ketchup (Autodesk Fusion 360 design; units mm, degrees)
Autodesk Fusion 360 part; units mm, degrees
sketch "Sketch1" plane through (0, 0, 0) normal (0, 0, 1) x (1, 0, 0)
  line L0 (0, 0) -> (-49, 0)
  line L1 (-49, 0) -> (-49, 88)
  line L2 (-49, 88) -> (0, 88)
  line L3 (0, 88) -> (0, 0)
  line L4 (-4, 4) -> (-45, 4)
  line L5 (-45, 4) -> (-45, 84)
  line L6 (-45, 84) -> (-4, 84)
  line L7 (-4, 84) -> (-4, 4)
  dimension "d1" = 49
  dimension "d2" = 88
  dimension "d3" = 4
  constraint horizontal L0
  constraint vertical L1
  constraint horizontal L2
  constraint vertical L3
  constraint coincident L0.start L3.end
  measures "d1" distance of L1.end L2.end
  measures "d2" distance of L0.start L2.end
extrude "Extrude1" add sketch "Sketch1" along normal blind 4 contours L0 L1 L2 L3 | L4 L5 L6 L7 makes body 1
extrude "Extrude2" add sketch "Sketch1" along normal blind 70 bodies 1
sketch "Sketch3" plane through (0, 0, 0) normal (0, -1, 0) x (1, 0, 0)
  line L0 (-49, 0) -> (0, 0)
  line L1 (0, 0) -> (0, 70)
  line L2 (0, 70) -> (-49, 70)
  line L3 (-49, 70) -> (-49, 0)
  line L4 (-43.8953, 12.2336) -> (-43.9282, 20.2336)
  line L5 (-43.9282, 20.2336) -> (-42.8695, 20.2379)
  line L6 (-42.8695, 20.2379) -> (-42.8532, 16.2707)
  line L7 (-42.8532, 16.2707) -> (-38.8968, 20.2542)
  line L8 (-38.8968, 20.2542) -> (-37.4617, 20.2601)
  line L9 (-37.4617, 20.2601) -> (-40.8044, 17.0049)
  line L10 (-40.8044, 17.0049) -> (-37.2815, 12.2608)
  line L11 (-37.2815, 12.2608) -> (-38.6784, 12.2551)
  line L12 (-38.6784, 12.2551) -> (-41.5436, 16.2924)
  line L13 (-41.5436, 16.2924) -> (-42.848, 15.0101)
  line L14 (-42.848, 15.0101) -> (-42.8367, 12.238)
  line L15 (-42.8367, 12.238) -> (-43.8953, 12.2336)
  line L16 (-32.5634, 14.1465) -> (-31.5479, 14.0252)
  spline S0 degree 2 poles (-31.5479, 14.0252) (-31.7843, 13.1347) (-32.4317, 12.6409) knots 0 0 0 1 1 1
  spline S1 degree 2 poles (-32.4317, 12.6409) (-33.079, 12.1471) (-34.0886, 12.143) knots 0 0 0 1 1 1
  spline S2 degree 2 poles (-34.0886, 12.143) (-35.3601, 12.1377) (-36.1082, 12.9178) knots 0 0 0 1 1 1
  spline S3 degree 2 poles (-36.1082, 12.9178) (-36.8562, 13.6978) (-36.8621, 15.1111) knots 0 0 0 1 1 1
  spline S4 degree 2 poles (-36.8621, 15.1111) (-36.8681, 16.5736) (-36.1183, 17.3843) knots 0 0 0 1 1 1
  spline S5 degree 2 poles (-36.1183, 17.3843) (-35.3686, 18.195) (-34.168, 18.2) knots 0 0 0 1 1 1
  spline S6 degree 2 poles (-34.168, 18.2) (-33.0057, 18.2048) (-32.2658, 17.4165) knots 0 0 0 1 1 1
  spline S7 degree 2 poles (-32.2658, 17.4165) (-31.5258, 16.6283) (-31.5199, 15.1931) knots 0 0 0 1 1 1
  spline S8 degree 2 poles (-31.5199, 15.1931) (-31.5196, 15.1058) (-31.5243, 14.9311) knots 0 0 0 1 1 1
  line L17 (-31.5243, 14.9311) -> (-35.8462, 14.9134)
  spline S9 degree 2 poles (-35.8462, 14.9134) (-35.7877, 13.9586) (-35.3, 13.4531) knots 0 0 0 1 1 1
  spline S10 degree 2 poles (-35.3, 13.4531) (-34.8122, 12.9476) (-34.0864, 12.9506) knots 0 0 0 1 1 1
  spline S11 degree 2 poles (-34.0864, 12.9506) (-33.5462, 12.9528) (-33.1654, 13.2382) knots 0 0 0 1 1 1
  spline S12 degree 2 poles (-33.1654, 13.2382) (-32.7846, 13.5235) (-32.5634, 14.1465) knots 0 0 0 1 1 1
  line L18 (-35.795, 15.7212) -> (-32.559, 15.7345)
  spline S13 degree 2 poles (-32.559, 15.7345) (-32.6275, 16.4655) (-32.9346, 16.8299) knots 0 0 0 1 1 1
  spline S14 degree 2 poles (-32.9346, 16.8299) (-33.4062, 17.3955) (-34.1538, 17.3924) knots 0 0 0 1 1 1
  spline S15 degree 2 poles (-34.1538, 17.3924) (-34.8305, 17.3896) (-35.2897, 16.9348) knots 0 0 0 1 1 1
  spline S16 degree 2 poles (-35.2897, 16.9348) (-35.749, 16.48) (-35.795, 15.7212) knots 0 0 0 1 1 1
  line L19 (-28.1664, 13.1768) -> (-28.021, 12.3098)
  spline S17 degree 2 poles (-28.021, 12.3098) (-28.4354, 12.2208) (-28.7628, 12.2194) knots 0 0 0 1 1 1
  spline S18 degree 2 poles (-28.7628, 12.2194) (-29.2976, 12.2172) (-29.5929, 12.3852) knots 0 0 0 1 1 1
  spline S19 degree 2 poles (-29.5929, 12.3852) (-29.8883, 12.5531) (-30.0095, 12.8282) knots 0 0 0 1 1 1
  spline S20 degree 2 poles (-30.0095, 12.8282) (-30.1307, 13.1033) (-30.1343, 13.9873) knots 0 0 0 1 1 1
  line L20 (-30.1343, 13.9873) -> (-30.148, 17.3215)
  line L21 (-30.148, 17.3215) -> (-30.8683, 17.3186)
  line L22 (-30.8683, 17.3186) -> (-30.8715, 18.0826)
  line L23 (-30.8715, 18.0826) -> (-30.1512, 18.0855)
  line L24 (-30.1512, 18.0855) -> (-30.1571, 19.5207)
  line L25 (-30.1571, 19.5207) -> (-29.1827, 20.1141)
  line L26 (-29.1827, 20.1141) -> (-29.1744, 18.0895)
  line L27 (-29.1744, 18.0895) -> (-28.1866, 18.0936)
  line L28 (-28.1866, 18.0936) -> (-28.1835, 17.3296)
  line L29 (-28.1835, 17.3296) -> (-29.1712, 17.3256)
  line L30 (-29.1712, 17.3256) -> (-29.1573, 13.9368)
  spline S21 degree 2 poles (-29.1573, 13.9368) (-29.1556, 13.5166) (-29.1032, 13.3967) knots 0 0 0 1 1 1
  spline S22 degree 2 poles (-29.1032, 13.3967) (-29.0509, 13.2769) (-28.9333, 13.2064) knots 0 0 0 1 1 1
  spline S23 degree 2 poles (-28.9333, 13.2064) (-28.8157, 13.136) (-28.5974, 13.1369) knots 0 0 0 1 1 1
  spline S24 degree 2 poles (-28.5974, 13.1369) (-28.4337, 13.1375) (-28.1664, 13.1768) knots 0 0 0 1 1 1
  line L31 (-23.4294, 14.4405) -> (-22.463, 14.319)
  spline S25 degree 2 poles (-22.463, 14.319) (-22.6172, 13.3197) (-23.267, 12.7522) knots 0 0 0 1 1 1
  spline S26 degree 2 poles (-23.267, 12.7522) (-23.9168, 12.1847) (-24.8663, 12.1808) knots 0 0 0 1 1 1
  spline S27 degree 2 poles (-24.8663, 12.1808) (-26.0559, 12.176) (-26.7821, 12.9506) knots 0 0 0 1 1 1
  spline S28 degree 2 poles (-26.7821, 12.9506) (-27.5084, 13.7253) (-27.5144, 15.1768) knots 0 0 0 1 1 1
  spline S29 degree 2 poles (-27.5144, 15.1768) (-27.5182, 16.1154) (-27.2101, 16.8206) knots 0 0 0 1 1 1
  spline S30 degree 2 poles (-27.2101, 16.8206) (-26.9019, 17.5259) (-26.2676, 17.8805) knots 0 0 0 1 1 1
  spline S31 degree 2 poles (-26.2676, 17.8805) (-25.6333, 18.235) (-24.8857, 18.2381) knots 0 0 0 1 1 1
  spline S32 degree 2 poles (-24.8857, 18.2381) (-23.9417, 18.242) (-23.3394, 17.767) knots 0 0 0 1 1 1
  spline S33 degree 2 poles (-23.3394, 17.767) (-22.7372, 17.292) (-22.5644, 16.4141) knots 0 0 0 1 1 1
  line L32 (-22.5644, 16.4141) -> (-23.5188, 16.2628)
  spline S34 degree 2 poles (-23.5188, 16.2628) (-23.6576, 16.8462) (-24.0053, 17.1394) knots 0 0 0 1 1 1
  spline S35 degree 2 poles (-24.0053, 17.1394) (-24.3531, 17.4327) (-24.8442, 17.4306) knots 0 0 0 1 1 1
  spline S36 degree 2 poles (-24.8442, 17.4306) (-25.5863, 17.4276) (-26.048, 16.8936) knots 0 0 0 1 1 1
  spline S37 degree 2 poles (-26.048, 16.8936) (-26.5097, 16.3597) (-26.5049, 15.2082) knots 0 0 0 1 1 1
  spline S38 degree 2 poles (-26.5049, 15.2082) (-26.5001, 14.0405) (-26.0505, 13.513) knots 0 0 0 1 1 1
  spline S39 degree 2 poles (-26.0505, 13.513) (-25.6008, 12.9855) (-24.8805, 12.9884) knots 0 0 0 1 1 1
  spline S40 degree 2 poles (-24.8805, 12.9884) (-24.3021, 12.9908) (-23.9161, 13.3471) knots 0 0 0 1 1 1
  spline S41 degree 2 poles (-23.9161, 13.3471) (-23.5301, 13.7034) (-23.4294, 14.4405) knots 0 0 0 1 1 1
  line L33 (-21.6145, 12.3252) -> (-21.6473, 20.3251)
  line L34 (-21.6473, 20.3251) -> (-20.6651, 20.3291)
  line L35 (-20.6651, 20.3291) -> (-20.6533, 17.4588)
  spline S42 degree 2 poles (-20.6533, 17.4588) (-19.969, 18.2583) (-18.9212, 18.2626) knots 0 0 0 1 1 1
  spline S43 degree 2 poles (-18.9212, 18.2626) (-18.2773, 18.2653) (-17.8015, 18.0135) knots 0 0 0 1 1 1
  spline S44 degree 2 poles (-17.8015, 18.0135) (-17.3257, 17.7617) (-17.1192, 17.315) knots 0 0 0 1 1 1
  spline S45 degree 2 poles (-17.1192, 17.315) (-16.9128, 16.8684) (-16.9093, 16.0171) knots 0 0 0 1 1 1
  line L36 (-16.9093, 16.0171) -> (-16.8942, 12.3446)
  line L37 (-16.8942, 12.3446) -> (-17.8764, 12.3405)
  line L38 (-17.8764, 12.3405) -> (-17.8915, 16.0131)
  spline S46 degree 2 poles (-17.8915, 16.0131) (-17.8945, 16.7498) (-18.2152, 17.0841) knots 0 0 0 1 1 1
  spline S47 degree 2 poles (-18.2152, 17.0841) (-18.5358, 17.4184) (-19.1197, 17.416) knots 0 0 0 1 1 1
  spline S48 degree 2 poles (-19.1197, 17.416) (-19.5562, 17.4142) (-19.94, 17.1861) knots 0 0 0 1 1 1
  spline S49 degree 2 poles (-19.94, 17.1861) (-20.3238, 16.9581) (-20.4859, 16.57) knots 0 0 0 1 1 1
  spline S50 degree 2 poles (-20.4859, 16.57) (-20.648, 16.1818) (-20.6452, 15.4997) knots 0 0 0 1 1 1
  line L39 (-20.6452, 15.4997) -> (-20.6322, 12.3292)
  line L40 (-20.6322, 12.3292) -> (-21.6145, 12.3252)
  line L41 (-11.6009, 12.3663) -> (-11.6044, 13.2176)
  spline S51 degree 2 poles (-11.6044, 13.2176) (-12.277, 12.2326) (-13.4394, 12.2278) knots 0 0 0 1 1 1
  spline S52 degree 2 poles (-13.4394, 12.2278) (-13.9523, 12.2257) (-14.3979, 12.4203) knots 0 0 0 1 1 1
  spline S53 degree 2 poles (-14.3979, 12.4203) (-14.8434, 12.6149) (-15.0602, 12.9115) knots 0 0 0 1 1 1
  spline S54 degree 2 poles (-15.0602, 12.9115) (-15.277, 13.208) (-15.3661, 13.6387) knots 0 0 0 1 1 1
  spline S55 degree 2 poles (-15.3661, 13.6387) (-15.4273, 13.9277) (-15.4298, 14.5552) knots 0 0 0 1 1 1
  line L42 (-15.4298, 14.5552) -> (-15.4446, 18.1459)
  line L43 (-15.4446, 18.1459) -> (-14.4623, 18.15)
  line L44 (-14.4623, 18.15) -> (-14.4491, 14.9358)
  spline S56 degree 2 poles (-14.4491, 14.9358) (-14.446, 14.1664) (-14.3849, 13.8992) knots 0 0 0 1 1 1
  spline S57 degree 2 poles (-14.3849, 13.8992) (-14.2905, 13.5122) (-13.9894, 13.2924) knots 0 0 0 1 1 1
  spline S58 degree 2 poles (-13.9894, 13.2924) (-13.6884, 13.0726) (-13.2464, 13.0744) knots 0 0 0 1 1 1
  spline S59 degree 2 poles (-13.2464, 13.0744) (-12.8044, 13.0762) (-12.4179, 13.3043) knots 0 0 0 1 1 1
  spline S60 degree 2 poles (-12.4179, 13.3043) (-12.0313, 13.5324) (-11.872, 13.9232) knots 0 0 0 1 1 1
  spline S61 degree 2 poles (-11.872, 13.9232) (-11.7126, 14.314) (-11.7156, 15.0562) knots 0 0 0 1 1 1
  line L45 (-11.7156, 15.0562) -> (-11.7284, 18.1612)
  line L46 (-11.7284, 18.1612) -> (-10.7461, 18.1652)
  line L47 (-10.7461, 18.1652) -> (-10.7223, 12.3699)
  line L48 (-10.7223, 12.3699) -> (-11.6009, 12.3663)
  line L49 (-9.1743, 10.1553) -> (-9.2073, 18.1716)
  line L50 (-9.2073, 18.1716) -> (-8.3123, 18.1752)
  line L51 (-8.3123, 18.1752) -> (-8.3092, 17.4222)
  spline S62 degree 2 poles (-8.3092, 17.4222) (-7.9945, 17.8655) (-7.5971, 18.0881) knots 0 0 0 1 1 1
  spline S63 degree 2 poles (-7.5971, 18.0881) (-7.1996, 18.3108) (-6.6321, 18.3131) knots 0 0 0 1 1 1
  spline S64 degree 2 poles (-6.6321, 18.3131) (-5.89, 18.3162) (-5.3209, 17.9365) knots 0 0 0 1 1 1
  spline S65 degree 2 poles (-5.3209, 17.9365) (-4.7518, 17.5568) (-4.4597, 16.8623) knots 0 0 0 1 1 1
  spline S66 degree 2 poles (-4.4597, 16.8623) (-4.1676, 16.1677) (-4.1642, 15.3382) knots 0 0 0 1 1 1
  spline S67 degree 2 poles (-4.1642, 15.3382) (-4.1606, 14.4487) (-4.4769, 13.7353) knots 0 0 0 1 1 1
  spline S68 degree 2 poles (-4.4769, 13.7353) (-4.7932, 13.0218) (-5.4001, 12.6401) knots 0 0 0 1 1 1
  spline S69 degree 2 poles (-5.4001, 12.6401) (-6.007, 12.2583) (-6.6782, 12.2556) knots 0 0 0 1 1 1
  spline S70 degree 2 poles (-6.6782, 12.2556) (-7.1693, 12.2536) (-7.5603, 12.4593) knots 0 0 0 1 1 1
  spline S71 degree 2 poles (-7.5603, 12.4593) (-7.9514, 12.6651) (-8.2037, 12.9806) knots 0 0 0 1 1 1
  line L52 (-8.2037, 12.9806) -> (-8.1921, 10.1593)
  line L53 (-8.1921, 10.1593) -> (-9.1743, 10.1553)
  spline S72 degree 2 poles (-8.3057, 15.2448) (-8.3011, 14.1261) (-7.846, 13.5932) knots 0 0 0 1 1 1
  spline S73 degree 2 poles (-7.846, 13.5932) (-7.3909, 13.0603) (-6.747, 13.0629) knots 0 0 0 1 1 1
  spline S74 degree 2 poles (-6.747, 13.0629) (-6.0921, 13.0656) (-5.6278, 13.6214) knots 0 0 0 1 1 1
  spline S75 degree 2 poles (-5.6278, 13.6214) (-5.1635, 14.1772) (-5.1683, 15.3396) knots 0 0 0 1 1 1
  spline S76 degree 2 poles (-5.1683, 15.3396) (-5.1729, 16.4473) (-5.6308, 16.9966) knots 0 0 0 1 1 1
  spline S77 degree 2 poles (-5.6308, 16.9966) (-6.0887, 17.5459) (-6.7217, 17.5433) knots 0 0 0 1 1 1
  spline S78 degree 2 poles (-6.7217, 17.5433) (-7.3493, 17.5407) (-7.8298, 16.9521) knots 0 0 0 1 1 1
  spline S79 degree 2 poles (-7.8298, 16.9521) (-8.3103, 16.3635) (-8.3057, 15.2448) knots 0 0 0 1 1 1
extrude "Extrude3" cut sketch "Sketch3" against normal blind 1 contours L4 L5 L6 L7 L8 L9 L10 L11 L12 L13 L14 L15 | L16 S0 S1 S2 S3 S4 S5 S6 S7 S8 L17 S9 S10 S11 S12 | L19 S17 S18 S19 S20 L20 L21 L22 L23 L24 L25 L26 L27 L28 L29 L30 S21 S22 S23 S24 | L31 S25 S26 S27 S28 S29 S30 S31 S32 S33 L32 S34 S35 S36 S37 S38 S39 S40 S41 | L33 L34 L35 S42 S43 S44 S45 L36 L37 L38 S46 S47 S48 S49 S50 L39 L40 | L41 S51 S52 S53 S54 S55 L42 L43 L44 S56 S57 S58 S59 S60 S61 L45 L46 L47 L48 | L49 L50 L51 S62 S63 S64 S65 S66 S67 S68 S69 S70 S71 L52 L53 bodies 1
sketch "Sketch5" plane through (0, 0, 70) normal (0, 0, 1) x (-1, 0, 0)
  line L0 (45, -84) -> (4, -84)
  line L1 (4, -84) -> (4, -4)
  line L2 (4, -4) -> (45, -4)
  line L3 (45, -4) -> (45, -84)
  line L4 (0, -88) -> (49, -88)
  line L5 (49, -88) -> (49, 0)
  line L6 (49, 0) -> (0, 0)
  line L7 (0, 0) -> (0, -88)
  line L8 (4, -4) -> (4, 0)
  line L9 (45, -4) -> (45, 0)
  constraint coincident L1.end L2.start
  constraint coincident L6 L8.end
  constraint perpendicular L6 L8
  constraint coincident L2.end L3.start
  constraint coincident L6 L9.end
  constraint perpendicular L6 L9
sketch "Sketch4" plane through (0, 0, 0) normal (0, -1, 0) x (1, 0, 0)
  line L0 (-49, 0) -> (0, 0)
  line L1 (0, 0) -> (0, 70)
  line L2 (0, 70) -> (-49, 70)
  line L3 (-49, 70) -> (-49, 0)
  spline S0 degree 2 poles (-45, 70) (-24.5, 0) (-4, 70) knots 0 0 0 8.378065 8.378065 8.378065 weights 1 1.091518 1
  line L4 (-24.5, 0) -> (-24.5, 70)
  spline S1 degree 2 poles (-20.4859, 16.57) (-20.648, 16.1818) (-20.6452, 15.4997) knots 0 0 0 1 1 1
  line L5 (-20.6452, 15.4997) -> (-20.6322, 12.3292)
  line L6 (-20.6322, 12.3292) -> (-21.6145, 12.3252)
  line L7 (-21.6145, 12.3252) -> (-21.6473, 20.3251)
  line L8 (-21.6473, 20.3251) -> (-20.6651, 20.3291)
  line L9 (-20.6651, 20.3291) -> (-20.6533, 17.4588)
  spline S2 degree 2 poles (-20.6533, 17.4588) (-19.969, 18.2583) (-18.9212, 18.2626) knots 0 0 0 1 1 1
  spline S3 degree 2 poles (-18.9212, 18.2626) (-18.2773, 18.2653) (-17.8015, 18.0135) knots 0 0 0 1 1 1
  spline S4 degree 2 poles (-17.8015, 18.0135) (-17.3257, 17.7617) (-17.1192, 17.315) knots 0 0 0 1 1 1
  spline S5 degree 2 poles (-17.1192, 17.315) (-16.9128, 16.8684) (-16.9093, 16.0171) knots 0 0 0 1 1 1
  line L10 (-16.9093, 16.0171) -> (-16.8942, 12.3446)
  line L11 (-16.8942, 12.3446) -> (-17.8764, 12.3405)
  line L12 (-17.8764, 12.3405) -> (-17.8915, 16.0131)
  spline S6 degree 2 poles (-17.8915, 16.0131) (-17.8945, 16.7498) (-18.2152, 17.0841) knots 0 0 0 1 1 1
  spline S7 degree 2 poles (-18.2152, 17.0841) (-18.5358, 17.4184) (-19.1197, 17.416) knots 0 0 0 1 1 1
  spline S8 degree 2 poles (-19.1197, 17.416) (-19.5562, 17.4142) (-19.94, 17.1861) knots 0 0 0 1 1 1
  spline S9 degree 2 poles (-19.94, 17.1861) (-20.3238, 16.9581) (-20.4859, 16.57) knots 0 0 0 1 1 1
  line L13 (-41.5436, 16.2924) -> (-42.848, 15.0101)
  line L14 (-42.848, 15.0101) -> (-42.8367, 12.238)
  line L15 (-42.8367, 12.238) -> (-43.8953, 12.2336)
  line L16 (-43.8953, 12.2336) -> (-43.9282, 20.2336)
  line L17 (-43.9282, 20.2336) -> (-42.8695, 20.2379)
  line L18 (-42.8695, 20.2379) -> (-42.8532, 16.2707)
  line L19 (-42.8532, 16.2707) -> (-38.8968, 20.2542)
  line L20 (-38.8968, 20.2542) -> (-37.4617, 20.2601)
  line L21 (-37.4617, 20.2601) -> (-40.8044, 17.0049)
  line L22 (-40.8044, 17.0049) -> (-37.2815, 12.2608)
  line L23 (-37.2815, 12.2608) -> (-38.6784, 12.2551)
  line L24 (-38.6784, 12.2551) -> (-41.5436, 16.2924)
  spline S10 degree 2 poles (-26.0505, 13.513) (-25.6008, 12.9855) (-24.8805, 12.9884) knots 0 0 0 1 1 1
  spline S11 degree 2 poles (-24.8805, 12.9884) (-24.3021, 12.9908) (-23.9161, 13.3471) knots 0 0 0 1 1 1
  spline S12 degree 2 poles (-23.9161, 13.3471) (-23.5301, 13.7034) (-23.4294, 14.4405) knots 0 0 0 1 1 1
  line L25 (-23.4294, 14.4405) -> (-22.463, 14.319)
  spline S13 degree 2 poles (-22.463, 14.319) (-22.6172, 13.3197) (-23.267, 12.7522) knots 0 0 0 1 1 1
  spline S14 degree 2 poles (-23.267, 12.7522) (-23.9168, 12.1847) (-24.8663, 12.1808) knots 0 0 0 1 1 1
  spline S15 degree 2 poles (-24.8663, 12.1808) (-26.0559, 12.176) (-26.7821, 12.9506) knots 0 0 0 1 1 1
  spline S16 degree 2 poles (-26.7821, 12.9506) (-27.5084, 13.7253) (-27.5144, 15.1768) knots 0 0 0 1 1 1
  spline S17 degree 2 poles (-27.5144, 15.1768) (-27.5182, 16.1154) (-27.2101, 16.8206) knots 0 0 0 1 1 1
  spline S18 degree 2 poles (-27.2101, 16.8206) (-26.9019, 17.5259) (-26.2676, 17.8805) knots 0 0 0 1 1 1
  spline S19 degree 2 poles (-26.2676, 17.8805) (-25.6333, 18.235) (-24.8857, 18.2381) knots 0 0 0 1 1 1
  spline S20 degree 2 poles (-24.8857, 18.2381) (-23.9417, 18.242) (-23.3394, 17.767) knots 0 0 0 1 1 1
  spline S21 degree 2 poles (-23.3394, 17.767) (-22.7372, 17.292) (-22.5644, 16.4141) knots 0 0 0 1 1 1
  line L26 (-22.5644, 16.4141) -> (-23.5188, 16.2628)
  spline S22 degree 2 poles (-23.5188, 16.2628) (-23.6576, 16.8462) (-24.0053, 17.1394) knots 0 0 0 1 1 1
  spline S23 degree 2 poles (-24.0053, 17.1394) (-24.3531, 17.4327) (-24.8442, 17.4306) knots 0 0 0 1 1 1
  spline S24 degree 2 poles (-24.8442, 17.4306) (-25.5863, 17.4276) (-26.048, 16.8936) knots 0 0 0 1 1 1
  spline S25 degree 2 poles (-26.048, 16.8936) (-26.5097, 16.3597) (-26.5049, 15.2082) knots 0 0 0 1 1 1
  spline S26 degree 2 poles (-26.5049, 15.2082) (-26.5001, 14.0405) (-26.0505, 13.513) knots 0 0 0 1 1 1
  line L27 (-11.7284, 18.1612) -> (-10.7461, 18.1652)
  line L28 (-10.7461, 18.1652) -> (-10.7223, 12.3699)
  line L29 (-10.7223, 12.3699) -> (-11.6009, 12.3663)
  line L30 (-11.6009, 12.3663) -> (-11.6044, 13.2176)
  spline S27 degree 2 poles (-11.6044, 13.2176) (-12.277, 12.2326) (-13.4394, 12.2278) knots 0 0 0 1 1 1
  spline S28 degree 2 poles (-13.4394, 12.2278) (-13.9523, 12.2257) (-14.3979, 12.4203) knots 0 0 0 1 1 1
  spline S29 degree 2 poles (-14.3979, 12.4203) (-14.8434, 12.6149) (-15.0602, 12.9115) knots 0 0 0 1 1 1
  spline S30 degree 2 poles (-15.0602, 12.9115) (-15.277, 13.208) (-15.3661, 13.6387) knots 0 0 0 1 1 1
  spline S31 degree 2 poles (-15.3661, 13.6387) (-15.4273, 13.9277) (-15.4298, 14.5552) knots 0 0 0 1 1 1
  line L31 (-15.4298, 14.5552) -> (-15.4446, 18.1459)
  line L32 (-15.4446, 18.1459) -> (-14.4623, 18.15)
  line L33 (-14.4623, 18.15) -> (-14.4491, 14.9358)
  spline S32 degree 2 poles (-14.4491, 14.9358) (-14.446, 14.1664) (-14.3849, 13.8992) knots 0 0 0 1 1 1
  spline S33 degree 2 poles (-14.3849, 13.8992) (-14.2905, 13.5122) (-13.9894, 13.2924) knots 0 0 0 1 1 1
  spline S34 degree 2 poles (-13.9894, 13.2924) (-13.6884, 13.0726) (-13.2464, 13.0744) knots 0 0 0 1 1 1
  spline S35 degree 2 poles (-13.2464, 13.0744) (-12.8044, 13.0762) (-12.4179, 13.3043) knots 0 0 0 1 1 1
  spline S36 degree 2 poles (-12.4179, 13.3043) (-12.0313, 13.5324) (-11.872, 13.9232) knots 0 0 0 1 1 1
  spline S37 degree 2 poles (-11.872, 13.9232) (-11.7126, 14.314) (-11.7156, 15.0562) knots 0 0 0 1 1 1
  line L34 (-11.7156, 15.0562) -> (-11.7284, 18.1612)
  spline S38 degree 2 poles (-35.3, 13.4531) (-34.8122, 12.9476) (-34.0864, 12.9506) knots 0 0 0 1 1 1
  spline S39 degree 2 poles (-34.0864, 12.9506) (-33.5462, 12.9528) (-33.1654, 13.2382) knots 0 0 0 1 1 1
  spline S40 degree 2 poles (-33.1654, 13.2382) (-32.7846, 13.5235) (-32.5634, 14.1465) knots 0 0 0 1 1 1
  line L35 (-32.5634, 14.1465) -> (-31.5479, 14.0252)
  spline S41 degree 2 poles (-31.5479, 14.0252) (-31.7843, 13.1347) (-32.4317, 12.6409) knots 0 0 0 1 1 1
  spline S42 degree 2 poles (-32.4317, 12.6409) (-33.079, 12.1471) (-34.0886, 12.143) knots 0 0 0 1 1 1
  spline S43 degree 2 poles (-34.0886, 12.143) (-35.3601, 12.1377) (-36.1082, 12.9178) knots 0 0 0 1 1 1
  spline S44 degree 2 poles (-36.1082, 12.9178) (-36.8562, 13.6978) (-36.8621, 15.1111) knots 0 0 0 1 1 1
  spline S45 degree 2 poles (-36.8621, 15.1111) (-36.8681, 16.5736) (-36.1183, 17.3843) knots 0 0 0 1 1 1
  spline S46 degree 2 poles (-36.1183, 17.3843) (-35.3686, 18.195) (-34.168, 18.2) knots 0 0 0 1 1 1
  spline S47 degree 2 poles (-34.168, 18.2) (-33.0057, 18.2048) (-32.2658, 17.4165) knots 0 0 0 1 1 1
  spline S48 degree 2 poles (-32.2658, 17.4165) (-31.5258, 16.6283) (-31.5199, 15.1931) knots 0 0 0 1 1 1
  spline S49 degree 2 poles (-31.5199, 15.1931) (-31.5196, 15.1058) (-31.5243, 14.9311) knots 0 0 0 1 1 1
  line L36 (-31.5243, 14.9311) -> (-35.8462, 14.9134)
  spline S50 degree 2 poles (-35.8462, 14.9134) (-35.7877, 13.9586) (-35.3, 13.4531) knots 0 0 0 1 1 1
  spline S51 degree 2 poles (-29.1032, 13.3967) (-29.0509, 13.2769) (-28.9333, 13.2064) knots 0 0 0 1 1 1
  spline S52 degree 2 poles (-28.9333, 13.2064) (-28.8157, 13.136) (-28.5974, 13.1369) knots 0 0 0 1 1 1
  spline S53 degree 2 poles (-28.5974, 13.1369) (-28.4337, 13.1375) (-28.1664, 13.1768) knots 0 0 0 1 1 1
  line L37 (-28.1664, 13.1768) -> (-28.021, 12.3098)
  spline S54 degree 2 poles (-28.021, 12.3098) (-28.4354, 12.2208) (-28.7628, 12.2194) knots 0 0 0 1 1 1
  spline S55 degree 2 poles (-28.7628, 12.2194) (-29.2976, 12.2172) (-29.5929, 12.3852) knots 0 0 0 1 1 1
  spline S56 degree 2 poles (-29.5929, 12.3852) (-29.8883, 12.5531) (-30.0095, 12.8282) knots 0 0 0 1 1 1
  spline S57 degree 2 poles (-30.0095, 12.8282) (-30.1307, 13.1033) (-30.1343, 13.9873) knots 0 0 0 1 1 1
  line L38 (-30.1343, 13.9873) -> (-30.148, 17.3215)
  line L39 (-30.148, 17.3215) -> (-30.8683, 17.3186)
  line L40 (-30.8683, 17.3186) -> (-30.8715, 18.0826)
  line L41 (-30.8715, 18.0826) -> (-30.1512, 18.0855)
  line L42 (-30.1512, 18.0855) -> (-30.1571, 19.5207)
  line L43 (-30.1571, 19.5207) -> (-29.1827, 20.1141)
  line L44 (-29.1827, 20.1141) -> (-29.1744, 18.0895)
  line L45 (-29.1744, 18.0895) -> (-28.1866, 18.0936)
  line L46 (-28.1866, 18.0936) -> (-28.1835, 17.3296)
  line L47 (-28.1835, 17.3296) -> (-29.1712, 17.3256)
  line L48 (-29.1712, 17.3256) -> (-29.1573, 13.9368)
  spline S58 degree 2 poles (-29.1573, 13.9368) (-29.1556, 13.5166) (-29.1032, 13.3967) knots 0 0 0 1 1 1
  spline S59 degree 2 poles (-7.5603, 12.4593) (-7.9514, 12.6651) (-8.2037, 12.9806) knots 0 0 0 1 1 1
  line L49 (-8.2037, 12.9806) -> (-8.1921, 10.1593)
  line L50 (-8.1921, 10.1593) -> (-9.1743, 10.1553)
  line L51 (-9.1743, 10.1553) -> (-9.2073, 18.1716)
  line L52 (-9.2073, 18.1716) -> (-8.3123, 18.1752)
  line L53 (-8.3123, 18.1752) -> (-8.3092, 17.4222)
  spline S60 degree 2 poles (-8.3092, 17.4222) (-7.9945, 17.8655) (-7.5971, 18.0881) knots 0 0 0 1 1 1
  spline S61 degree 2 poles (-7.5971, 18.0881) (-7.1996, 18.3108) (-6.6321, 18.3131) knots 0 0 0 1 1 1
  spline S62 degree 2 poles (-6.6321, 18.3131) (-5.89, 18.3162) (-5.3209, 17.9365) knots 0 0 0 1 1 1
  spline S63 degree 2 poles (-5.3209, 17.9365) (-4.7518, 17.5568) (-4.4597, 16.8623) knots 0 0 0 1 1 1
  spline S64 degree 2 poles (-4.4597, 16.8623) (-4.1676, 16.1677) (-4.1642, 15.3382) knots 0 0 0 1 1 1
  spline S65 degree 2 poles (-4.1642, 15.3382) (-4.1606, 14.4487) (-4.4769, 13.7353) knots 0 0 0 1 1 1
  spline S66 degree 2 poles (-4.4769, 13.7353) (-4.7932, 13.0218) (-5.4001, 12.6401) knots 0 0 0 1 1 1
  spline S67 degree 2 poles (-5.4001, 12.6401) (-6.007, 12.2583) (-6.6782, 12.2556) knots 0 0 0 1 1 1
  spline S68 degree 2 poles (-6.6782, 12.2556) (-7.1693, 12.2536) (-7.5603, 12.4593) knots 0 0 0 1 1 1
  point P0 (-4, 70)
  point P1 (-45, 70)
  constraint coincident L2 P0
  constraint coincident L2 P1
  constraint coincident P0 S0.end
  constraint coincident P1 S0.start
  constraint midpoint L0 L4.start
  constraint midpoint L2 L4.end
extrude "Extrude4" cut sketch "Sketch4" against normal blind 66 contours L2 S0 L4 | L2 S0 L4 bodies 1
extrude "Extrude1'" add 7 faces at (-38.9214, 1, 13.8403) (-33.3098, 1, 15.193) (-29.4876, 1, 15.0832) (-26.8229, 1, 14.866) (-21.2999, 1, 16.1494) (-11.0614, 1, 15.1971) (-8.8813, 1, 14.3177) along direction (0, -1, 0) blind 1 separate body on bodies 1 makes body 2 at (-11.0614, 1, 15.1971) makes body 3 at (-26.8229, 1, 14.866) makes body 4 at (-33.3098, 1, 15.193) makes body 5 at (-38.9214, 1, 13.8403) makes body 6 at (-29.4876, 1, 15.0832) makes body 7 at (-21.2999, 1, 16.1494) makes body 8 at (-8.8813, 1, 14.3177) in component "Component"
component "Component" placed x (1, 0, 0) y (0, 1, 0) z (0, 0, 1) at (0, 0, 0)
equation "d1 = 41 mm + 8 mm"
